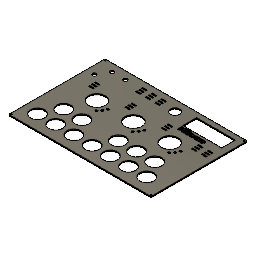
ArpeggioCase (Autodesk Fusion 360 design; units mm, degrees)
Autodesk Fusion 360 part; units mm, degrees
note: some values were not read from the file. Chosen so that the rebuilt part matches the saved one: a direction.
sketch "Sketch1" plane through (0, 0, 0) normal (0, 1, 0) x (1, 0, 0) in component "box"
  line L0 (130, 90) -> (-130, 90)
  line L1 (-130, 90) -> (-130, -90)
  line L2 (-130, -90) -> (130, -90)
  line L3 (130, -90) -> (130, 90)
  line L4 (130, 90) -> (-130, -90) construction
  line L5 (-130, 90) -> (130, -90) construction
  dimension "d1" = 260
  dimension "d2" = 180
extrude "Extrude1" add sketch "Sketch1" along normal blind 2 in component "box"
sketch "Sketch2" plane through (0, 2, 0) normal (0, 1, 0) x (-1, 0, 0) in component "box"
  line L0 (-130, 90) -> (-130, -90)
  line L1 (-130, -90) -> (130, -90)
  line L2 (130, -90) -> (130, 90)
  line L3 (130, 90) -> (-130, 90)
  circle A0 centre (107, 62) radius 13
  circle A1 centre (107, 62) radius 13
  circle A2 centre (73, 62) radius 13
  circle A3 centre (39, 62) radius 13
  circle A4 centre (5, 62) radius 13
  circle A5 centre (-29, 62) radius 13
  circle A6 centre (-63, 62) radius 13
  circle A7 centre (-97, 62) radius 13
  circle A8 centre (90, 30) radius 13
  circle A9 centre (56, 30) radius 13
  circle A10 centre (-12, 30) radius 13
  circle A11 centre (-46, 30) radius 13
  circle A12 centre (-80, 30) radius 13
  circle A13 centre (73, -15) radius 15.5
  circle A14 centre (73, -15) radius 15.5
  circle A15 centre (5, -15) radius 15.5
  circle A16 centre (-63, -15) radius 15.5
  line L4 (-120, -55) -> (-48, -55)
  line L5 (-48, -55) -> (-48, -80)
  line L6 (-48, -80) -> (-120, -80)
  line L7 (-120, -80) -> (-120, -55)
  line L8 (-120, -55) -> (-48, -80) construction
  line L9 (-48, -55) -> (-120, -80) construction
  circle A17 centre (105, -75) radius 3.5
  circle A18 centre (80, -75) radius 3.5
  circle A19 centre (-18, -70) radius 8.5
  dimension "d5" = 26
  dimension "d10" = 23
  dimension "d11" = 28
  dimension "d12" = 26
  dimension "d13" = 26
  dimension "d14" = 26
  dimension "d15" = 26
  dimension "d16" = 26
  dimension "d17" = 26
  dimension "d18" = 26
  dimension "d33" = 26
  dimension "d34" = 40
  dimension "d35" = 60
  dimension "d36" = 26
  dimension "d37" = 26
  dimension "d38" = 26
  dimension "d39" = 26
  dimension "d41" = 31
  dimension "d42" = 34
  dimension "d43" = 34
  dimension "d44" = 34
  dimension "d45" = 34
  dimension "d46" = 34
  dimension "d47" = 34
  dimension "d48" = 45
  dimension "d49" = 31
  dimension "d50" = 31
  dimension "d51" = 31
  dimension "d52" = 72
  dimension "d53" = 25
  dimension "d54" = 10
  dimension "d55" = 10
  dimension "d56" = 7
  dimension "d57" = 25
  dimension "d58" = 15
  dimension "d59" = 7
  dimension "d60" = 25
  dimension "d62" = 17
  dimension "d63" = 30
  dimension "d64" = 20
  measures "d5" diameter of A0
  measures "d12" diameter of A1
  measures "d13" diameter of A2
  measures "d14" diameter of A3
  measures "d15" diameter of A4
  measures "d16" diameter of A5
  measures "d17" diameter of A6
  measures "d18" diameter of A7
  measures "d33" diameter of A8
  measures "d36" diameter of A9
  measures "d37" diameter of A10
  measures "d38" diameter of A11
  measures "d39" diameter of A12
  measures "d41" diameter of A13
  measures "d44" distance of origin
  measures "d45" distance of origin
  measures "d48" distance of origin
  measures "d49" diameter of A14
  measures "d50" diameter of A15
  measures "d51" diameter of A16
  measures "d54" distance of L0 L7
  measures "d55" distance of L1 L6
  measures "d56" diameter of A17
  measures "d59" diameter of A18
  measures "d62" diameter of A19
extrude "Extrude9" cut sketch "Sketch2" against normal blind 2 contours A0 A1 | A2 | A3 | A4 | A5 | A6 | A7 | A8 | A9 | A10 | A11 | A12 | A13 A14 | A15 | A16 | L4 L5 L6 L7 | A17 | A18 | A19 in component "box"
sketch "Sketch1 (2)" plane through (0, 2, 0) normal (0, 1, 0) x (-1, 0, 0)
  line L0 (-48, -55) -> (-48, -80)
  line L1 (-48, -80) -> (-120, -80)
  line L2 (-120, -80) -> (-120, -55)
  line L3 (-120, -55) -> (-48, -55)
  circle A0 centre (73, -15) radius 15.5
  circle A1 centre (56, 30) radius 13
  circle A2 centre (-29, 62) radius 13
  circle A3 centre (107, 62) radius 13
  circle A4 centre (5, 62) radius 13
  circle A5 centre (90, 30) radius 13
  circle A6 centre (-80, 30) radius 13
  circle A7 centre (-18, -70) radius 8.5
  circle A8 centre (80, -75) radius 3.5
  circle A9 centre (5, -15) radius 15.5
  circle A10 centre (-12, 30) radius 13
  circle A11 centre (-63, 62) radius 13
  circle A12 centre (73, 62) radius 13
  circle A13 centre (39, 62) radius 13
  circle A14 centre (-97, 62) radius 13
  circle A15 centre (-46, 30) radius 13
  circle A16 centre (-63, -15) radius 15.5
  circle A17 centre (105, -75) radius 3.5
  line L4 (130, -90) -> (130, 90)
  line L5 (130, 90) -> (-130, 90)
  line L6 (-130, 90) -> (-130, -90)
  line L7 (-130, -90) -> (130, -90)
  line L8 (96, -43.5014) -> (104, -43.5014)
  line L9 (104, -43.5014) -> (104, -41.5014)
  line L10 (104, -41.5014) -> (96, -41.5014)
  line L11 (96, -41.5014) -> (96, -43.5014)
  line L12 (96, -43.5014) -> (104, -41.5014) construction
  line L13 (104, -43.5014) -> (96, -41.5014) construction
  line L14 (96, -32.5014) -> (104, -32.5014)
  line L15 (104, -32.5014) -> (104, -30.5014)
  line L16 (96, -30.5014) -> (96, -32.5014)
  line L17 (104, -30.5014) -> (96, -30.5014)
  line L18 (96, -32.5014) -> (104, -30.5014) construction
  line L19 (104, -32.5014) -> (96, -30.5014) construction
  line L20 (96, -36.0014) -> (96, -38.0014)
  line L21 (104, -38.0014) -> (96, -36.0014) construction
  line L22 (104, -36.0014) -> (96, -36.0014)
  line L23 (96, -38.0014) -> (104, -38.0014)
  line L24 (96, -38.0014) -> (104, -36.0014) construction
  line L25 (104, -38.0014) -> (104, -36.0014)
  line L26 (28, -38.0014) -> (36, -38.0014)
  line L27 (36, -30.5014) -> (28, -30.5014)
  line L28 (36, -38.0014) -> (36, -36.0014)
  line L29 (28, -43.5014) -> (36, -41.5014) construction
  line L30 (28, -32.5014) -> (36, -30.5014) construction
  line L31 (36, -32.5014) -> (28, -30.5014) construction
  line L32 (28, -36.0014) -> (28, -38.0014)
  line L33 (28, -30.5014) -> (28, -32.5014)
  line L34 (36, -43.5014) -> (36, -41.5014)
  line L35 (36, -43.5014) -> (28, -41.5014) construction
  line L36 (28, -38.0014) -> (36, -36.0014) construction
  line L37 (36, -32.5014) -> (36, -30.5014)
  line L38 (36, -41.5014) -> (28, -41.5014)
  line L39 (36, -38.0014) -> (28, -36.0014) construction
  line L40 (28, -32.5014) -> (36, -32.5014)
  line L41 (28, -43.5014) -> (36, -43.5014)
  line L42 (36, -36.0014) -> (28, -36.0014)
  line L43 (28, -41.5014) -> (28, -43.5014)
  line L44 (-32, -38.0014) -> (-32, -36.0014)
  line L45 (-40, -43.5014) -> (-32, -43.5014)
  line L46 (-40, -32.5014) -> (-32, -32.5014)
  line L47 (-32, -38.0014) -> (-40, -36.0014) construction
  line L48 (-40, -43.5014) -> (-32, -41.5014) construction
  line L49 (-32, -30.5014) -> (-40, -30.5014)
  line L50 (-40, -38.0014) -> (-32, -38.0014)
  line L51 (-40, -38.0014) -> (-32, -36.0014) construction
  line L52 (-40, -30.5014) -> (-40, -32.5014)
  line L53 (-32, -32.5014) -> (-32, -30.5014)
  line L54 (-40, -32.5014) -> (-32, -30.5014) construction
  line L55 (-32, -43.5014) -> (-32, -41.5014)
  line L56 (-32, -41.5014) -> (-40, -41.5014)
  line L57 (-40, -41.5014) -> (-40, -43.5014)
  line L58 (-32, -43.5014) -> (-40, -41.5014) construction
  line L59 (-32, -36.0014) -> (-40, -36.0014)
  line L60 (-32, -32.5014) -> (-40, -30.5014) construction
  line L61 (-40, -36.0014) -> (-40, -38.0014)
  circle A18 centre (48.684, -11.0058) radius 2
  circle A19 centre (52, -4) radius 2
  circle A20 centre (57, 2) radius 2
  circle A21 centre (-16, -4) radius 2
  circle A22 centre (-11, 2) radius 2
  circle A23 centre (-19.316, -11.0058) radius 2
  circle A24 centre (-87.316, -11.0058) radius 2
  circle A25 centre (-84, -4) radius 2
  circle A26 centre (-79, 2) radius 2
  line L62 (-120, -27.5014) -> (-112, -25.5014) construction
  line L63 (-112, -38.5014) -> (-120, -36.5014) construction
  line L64 (-112, -31.0014) -> (-120, -31.0014)
  line L65 (-112, -36.5014) -> (-120, -36.5014)
  line L66 (-112, -27.5014) -> (-112, -25.5014)
  line L67 (-112, -38.5014) -> (-112, -36.5014)
  line L68 (-112, -27.5014) -> (-120, -25.5014) construction
  line L69 (-120, -36.5014) -> (-120, -38.5014)
  line L70 (-120, -33.0014) -> (-112, -31.0014) construction
  line L71 (-120, -27.5014) -> (-112, -27.5014)
  line L72 (-120, -38.5014) -> (-112, -36.5014) construction
  line L73 (-112, -33.0014) -> (-120, -31.0014) construction
  line L74 (-120, -25.5014) -> (-120, -27.5014)
  line L75 (-120, -31.0014) -> (-120, -33.0014)
  line L76 (-112, -33.0014) -> (-112, -31.0014)
  line L77 (-112, -25.5014) -> (-120, -25.5014)
  line L78 (-120, -38.5014) -> (-112, -38.5014)
  line L79 (-120, -33.0014) -> (-112, -33.0014)
  line L80 (-101.4634, -27.3193) -> (-93.4634, -27.3193)
  line L81 (-101.4634, -25.3193) -> (-101.4634, -27.3193)
  line L82 (-93.4634, -36.3193) -> (-101.4634, -36.3193)
  line L83 (-101.4634, -36.3193) -> (-101.4634, -38.3193)
  line L84 (-93.4634, -38.3193) -> (-101.4634, -36.3193) construction
  line L85 (-93.4634, -30.8193) -> (-101.4634, -30.8193)
  line L86 (-93.4634, -27.3193) -> (-101.4634, -25.3193) construction
  line L87 (-101.4634, -32.8193) -> (-93.4634, -30.8193) construction
  line L88 (-93.4634, -25.3193) -> (-101.4634, -25.3193)
  line L89 (-101.4634, -38.3193) -> (-93.4634, -36.3193) construction
  line L90 (-101.4634, -30.8193) -> (-101.4634, -32.8193)
  line L91 (-101.4634, -27.3193) -> (-93.4634, -25.3193) construction
  line L92 (-93.4634, -27.3193) -> (-93.4634, -25.3193)
  line L93 (-93.4634, -38.3193) -> (-93.4634, -36.3193)
  line L94 (-93.4634, -32.8193) -> (-93.4634, -30.8193)
  line L95 (-101.4634, -38.3193) -> (-93.4634, -38.3193)
  line L96 (-93.4634, -32.8193) -> (-101.4634, -30.8193) construction
  line L97 (-101.4634, -32.8193) -> (-93.4634, -32.8193)
  line L98 (43, -73.0014) -> (51, -73.0014)
  line L99 (51, -67.5014) -> (43, -65.5014) construction
  line L100 (51, -71.0014) -> (43, -71.0014)
  line L101 (51, -76.5014) -> (43, -76.5014)
  line L102 (43, -76.5014) -> (43, -78.5014)
  line L103 (43, -65.5014) -> (43, -67.5014)
  line L104 (43, -73.0014) -> (51, -71.0014) construction
  line L105 (51, -67.5014) -> (51, -65.5014)
  line L106 (43, -67.5014) -> (51, -67.5014)
  line L107 (51, -73.0014) -> (51, -71.0014)
  line L108 (51, -65.5014) -> (43, -65.5014)
  line L109 (43, -71.0014) -> (43, -73.0014)
  line L110 (51, -78.5014) -> (51, -76.5014)
  line L111 (43, -78.5014) -> (51, -78.5014)
  line L112 (51, -78.5014) -> (43, -76.5014) construction
  line L113 (43, -78.5014) -> (51, -76.5014) construction
  line L114 (43, -67.5014) -> (51, -65.5014) construction
  line L115 (51, -73.0014) -> (43, -71.0014) construction
  line L116 (25, -65.5014) -> (25, -67.5014)
  line L117 (25, -73.0014) -> (33, -73.0014)
  line L118 (33, -71.0014) -> (25, -71.0014)
  line L119 (33, -76.5014) -> (25, -76.5014)
  line L120 (33, -67.5014) -> (25, -65.5014) construction
  line L121 (25, -76.5014) -> (25, -78.5014)
  line L122 (25, -73.0014) -> (33, -71.0014) construction
  line L123 (33, -67.5014) -> (33, -65.5014)
  line L124 (25, -67.5014) -> (33, -67.5014)
  line L125 (25, -78.5014) -> (33, -78.5014)
  line L126 (25, -78.5014) -> (33, -76.5014) construction
  line L127 (33, -78.5014) -> (25, -76.5014) construction
  line L128 (25, -67.5014) -> (33, -65.5014) construction
  line L129 (33, -73.0014) -> (25, -71.0014) construction
  line L130 (33, -73.0014) -> (33, -71.0014)
  line L131 (33, -65.5014) -> (25, -65.5014)
  line L132 (33, -78.5014) -> (33, -76.5014)
  line L133 (25, -71.0014) -> (25, -73.0014)
  line L134 (7, -67.5014) -> (15, -65.5014) construction
  line L135 (7, -67.5014) -> (15, -67.5014)
  line L136 (15, -65.5014) -> (7, -65.5014)
  line L137 (7, -73.0014) -> (15, -73.0014)
  line L138 (7, -71.0014) -> (7, -73.0014)
  line L139 (15, -71.0014) -> (7, -71.0014)
  line L140 (15, -76.5014) -> (7, -76.5014)
  line L141 (7, -73.0014) -> (15, -71.0014) construction
  line L142 (15, -78.5014) -> (15, -76.5014)
  line L143 (15, -67.5014) -> (15, -65.5014)
  line L144 (15, -73.0014) -> (7, -71.0014) construction
  line L145 (7, -78.5014) -> (15, -76.5014) construction
  line L146 (7, -78.5014) -> (15, -78.5014)
  line L147 (15, -78.5014) -> (7, -76.5014) construction
  line L148 (15, -73.0014) -> (15, -71.0014)
  line L149 (7, -65.5014) -> (7, -67.5014)
  line L150 (7, -76.5014) -> (7, -78.5014)
  line L151 (15, -67.5014) -> (7, -65.5014) construction
  dimension "d67" = 8
  dimension "d68" = 2
  dimension "d69" = 8
  dimension "d70" = 2
  dimension "d71" = 13
  dimension "d72" = 8
  dimension "d73" = 2
  dimension "d74" = 6.5
  dimension "d75" = 8
  dimension "d76" = 2
  dimension "d77" = 8
  dimension "d78" = 2
  dimension "d79" = 13
  dimension "d80" = 8
  dimension "d81" = 2
  dimension "d82" = 6.5
  dimension "d83" = 8
  dimension "d84" = 2
  dimension "d85" = 8
  dimension "d86" = 2
  dimension "d87" = 13
  dimension "d88" = 8
  dimension "d89" = 2
  dimension "d90" = 6.5
  dimension "d92" = 23
  dimension "d93" = 23
  dimension "d94" = 23
  dimension "d97" = 4
  dimension "d98" = 4
  dimension "d99" = 4
  dimension "d100" = 4
  dimension "d101" = 4
  dimension "d102" = 4
  dimension "d103" = 4
  dimension "d104" = 4
  dimension "d105" = 4
  dimension "d106" = 8
  dimension "d107" = 2
  dimension "d108" = 8
  dimension "d109" = 2
  dimension "d110" = 13
  dimension "d111" = 8
  dimension "d112" = 2
  dimension "d113" = 6.5
  dimension "d114" = 8
  dimension "d115" = 2
  dimension "d116" = 8
  dimension "d117" = 2
  dimension "d118" = 13
  dimension "d119" = 8
  dimension "d120" = 2
  dimension "d121" = 6.5
  dimension "d122" = 8
  dimension "d123" = 2
  dimension "d124" = 8
  dimension "d125" = 2
  dimension "d126" = 13
  dimension "d127" = 8
  dimension "d128" = 2
  dimension "d129" = 6.5
  dimension "d130" = 8
  dimension "d131" = 2
  dimension "d132" = 8
  dimension "d133" = 2
  dimension "d134" = 13
  dimension "d135" = 8
  dimension "d136" = 2
  dimension "d137" = 6.5
  dimension "d138" = 8
  dimension "d139" = 2
  dimension "d140" = 8
  dimension "d141" = 2
  dimension "d142" = 13
  dimension "d143" = 8
  dimension "d144" = 2
  dimension "d145" = 6.5
  dimension "d146" = 10
  dimension "d147" = 10
  measures "d92" distance of origin
  measures "d93" distance of origin
  measures "d94" distance of origin
  measures "d97" diameter of A18
  measures "d98" diameter of A19
  measures "d99" diameter of A20
  measures "d100" diameter of A23
  measures "d101" diameter of A21
  measures "d102" diameter of A22
  measures "d103" diameter of A24
  measures "d104" diameter of A25
  measures "d105" diameter of A26
  measures "d147" distance of origin
extrude "Extrude10" cut sketch "Sketch1 (2)" against normal blind 2 contours L8 L9 L10 L11 | L14 L15 L16 L17 | L20 L22 L23 L25 | L26 L28 L32 L42 | L27 L33 L37 L40 | L34 L38 L41 L43 | L44 L50 L59 L61 | L45 L55 L56 L57 | L46 L49 L52 L53 | A18 | A19 | A20 | A21 | A22 | A23 | A24 | A25 | A26 | L64 L75 L76 L79 | L65 L67 L69 L78 | L66 L71 L74 L77 | L80 L81 L88 L92 | L82 L83 L93 L95 | L85 L90 L94 L97 | L98 L100 L107 L109 | L101 L102 L110 L111 | L103 L105 L106 L108 | L116 L123 L124 L131 | L117 L118 L130 L133 | L119 L121 L125 L132 | L135 L136 L143 L149 | L137 L138 L139 L148 | L140 L142 L146 L150 in component "box"
extrude "Extrude11" add 1 faces at (130, 0.6667, 30) along direction (1, 0, 0) blind 3 in component "box"
extrude "Extrude12" add 1 faces at (-130, 0.6667, -30) along direction (-1, 0, 0) blind 3 in component "box"
hole "Hole1" at (-130, 2, 87) direction (0, -1, 0) diameter 1.875 depth 2 tip angle 118 in component "box"
thread "Thread1" "ISO Metric profile 2.3 M2.3x0.45 6H" in component "box"
pattern_linear "R-Pattern1" count 2 spacing 174 along (0, 0, -1) count 2 spacing 260 along (1, 0, 0) of "Hole1" in component "box"
sketch "Sketch2 (2)" plane through (0, 37.5554, 0) normal (0, 1, 0) x (-1, 0, 0)
  circle A0 centre (-43.4219, 26.2013) radius 0.9377
  circle A1 centre (-43.4219, 200.2013) radius 0.9377
  circle A2 centre (216.5781, 26.2013) radius 0.9377
  circle A3 centre (216.5781, 200.2013) radius 0.9377
  line L0 (101.5781, 45.6998) -> (93.5781, 45.6998)
  line L1 (93.5781, 45.6998) -> (93.5781, 47.6998)
  line L2 (93.5781, 47.6998) -> (101.5781, 47.6998)
  line L3 (101.5781, 47.6998) -> (101.5781, 45.6998)
  circle A4 centre (7.5781, 115.2013) radius 2
  circle A5 centre (138.5781, 109.2013) radius 2
  circle A6 centre (67.2621, 102.1955) radius 2
  line L4 (-14.8853, 87.8819) -> (-6.8853, 87.8819)
  line L5 (-6.8853, 87.8819) -> (-6.8853, 85.8819)
  line L6 (-6.8853, 85.8819) -> (-14.8853, 85.8819)
  line L7 (-14.8853, 85.8819) -> (-14.8853, 87.8819)
  line L8 (137.5781, 40.1998) -> (129.5781, 40.1998)
  line L9 (129.5781, 40.1998) -> (129.5781, 42.1998)
  line L10 (129.5781, 42.1998) -> (137.5781, 42.1998)
  line L11 (137.5781, 42.1998) -> (137.5781, 40.1998)
  line L12 (54.5781, 69.6998) -> (46.5781, 69.6998)
  line L13 (46.5781, 69.6998) -> (46.5781, 71.6998)
  line L14 (46.5781, 71.6998) -> (54.5781, 71.6998)
  line L15 (54.5781, 71.6998) -> (54.5781, 69.6998)
  line L16 (190.5781, 69.6998) -> (182.5781, 69.6998)
  line L17 (182.5781, 69.6998) -> (182.5781, 71.6998)
  line L18 (182.5781, 71.6998) -> (190.5781, 71.6998)
  line L19 (190.5781, 71.6998) -> (190.5781, 69.6998)
  line L20 (182.5781, 77.1998) -> (190.5781, 77.1998)
  line L21 (190.5781, 77.1998) -> (190.5781, 75.1998)
  line L22 (190.5781, 75.1998) -> (182.5781, 75.1998)
  line L23 (182.5781, 75.1998) -> (182.5781, 77.1998)
  line L24 (122.5781, 69.6998) -> (114.5781, 69.6998)
  line L25 (114.5781, 69.6998) -> (114.5781, 71.6998)
  line L26 (114.5781, 71.6998) -> (122.5781, 71.6998)
  line L27 (122.5781, 71.6998) -> (122.5781, 69.6998)
  line L28 (137.5781, 36.6998) -> (137.5781, 34.6998)
  line L29 (137.5781, 34.6998) -> (129.5781, 34.6998)
  line L30 (129.5781, 34.6998) -> (129.5781, 36.6998)
  line L31 (129.5781, 36.6998) -> (137.5781, 36.6998)
  line L32 (-6.8852, 82.3819) -> (-6.8852, 80.3819)
  line L33 (-6.8852, 80.3819) -> (-14.8852, 80.3819)
  line L34 (-14.8852, 80.3819) -> (-14.8852, 82.3819)
  line L35 (-14.8852, 82.3819) -> (-6.8852, 82.3819)
  line L36 (-25.4219, 76.6998) -> (-25.4219, 74.6998)
  line L37 (-25.4219, 74.6998) -> (-33.4219, 74.6998)
  line L38 (-33.4219, 74.6998) -> (-33.4219, 76.6998)
  line L39 (-33.4219, 76.6998) -> (-25.4219, 76.6998)
  circle A7 centre (143.5781, 115.2013) radius 2
  circle A8 centre (2.5781, 109.2013) radius 2
  line L40 (111.5781, 45.6998) -> (111.5781, 47.6998)
  line L41 (111.5781, 47.6998) -> (119.5781, 47.6998)
  line L42 (119.5781, 47.6998) -> (119.5781, 45.6998)
  line L43 (119.5781, 45.6998) -> (111.5781, 45.6998)
  line L44 (93.5781, 42.1998) -> (101.5781, 42.1998)
  line L45 (101.5781, 42.1998) -> (101.5781, 40.1998)
  line L46 (101.5781, 40.1998) -> (93.5781, 40.1998)
  line L47 (93.5781, 40.1998) -> (93.5781, 42.1998)
  line L48 (111.5781, 36.6998) -> (119.5781, 36.6998)
  line L49 (119.5781, 36.6998) -> (119.5781, 34.6998)
  line L50 (119.5781, 34.6998) -> (111.5781, 34.6998)
  line L51 (111.5781, 34.6998) -> (111.5781, 36.6998)
  circle A9 centre (135.2621, 102.1955) radius 2
  circle A10 centre (70.5781, 109.2013) radius 2
  line L52 (-33.4219, 85.6998) -> (-33.4219, 87.6998)
  line L53 (-33.4219, 87.6998) -> (-25.4219, 87.6998)
  line L54 (-25.4219, 87.6998) -> (-25.4219, 85.6998)
  line L55 (-25.4219, 85.6998) -> (-33.4219, 85.6998)
  line L56 (129.5781, 45.6998) -> (129.5781, 47.6998)
  line L57 (129.5781, 47.6998) -> (137.5781, 47.6998)
  line L58 (137.5781, 47.6998) -> (137.5781, 45.6998)
  line L59 (137.5781, 45.6998) -> (129.5781, 45.6998)
  line L60 (54.5781, 75.1998) -> (46.5781, 75.1998)
  line L61 (46.5781, 75.1998) -> (46.5781, 77.1998)
  line L62 (46.5781, 77.1998) -> (54.5781, 77.1998)
  line L63 (54.5781, 77.1998) -> (54.5781, 75.1998)
  line L64 (122.5781, 82.6998) -> (122.5781, 80.6998)
  line L65 (122.5781, 80.6998) -> (114.5781, 80.6998)
  line L66 (114.5781, 80.6998) -> (114.5781, 82.6998)
  line L67 (114.5781, 82.6998) -> (122.5781, 82.6998)
  line L68 (182.5781, 80.6998) -> (182.5781, 82.6998)
  line L69 (182.5781, 82.6998) -> (190.5781, 82.6998)
  line L70 (190.5781, 82.6998) -> (190.5781, 80.6998)
  line L71 (190.5781, 80.6998) -> (182.5781, 80.6998)
  line L72 (114.5781, 75.1998) -> (114.5781, 77.1998)
  line L73 (114.5781, 77.1998) -> (122.5781, 77.1998)
  line L74 (122.5781, 77.1998) -> (122.5781, 75.1998)
  line L75 (122.5781, 75.1998) -> (114.5781, 75.1998)
  line L76 (46.5781, 82.6998) -> (54.5781, 82.6998)
  line L77 (54.5781, 82.6998) -> (54.5781, 80.6998)
  line L78 (54.5781, 80.6998) -> (46.5781, 80.6998)
  line L79 (46.5781, 80.6998) -> (46.5781, 82.6998)
  line L80 (-6.8852, 76.8819) -> (-6.8852, 74.8819)
  line L81 (-6.8852, 74.8819) -> (-14.8852, 74.8819)
  line L82 (-14.8852, 74.8819) -> (-14.8852, 76.8819)
  line L83 (-14.8852, 76.8819) -> (-6.8852, 76.8819)
  line L84 (-25.4219, 82.1998) -> (-25.4219, 80.1998)
  line L85 (-25.4219, 80.1998) -> (-33.4219, 80.1998)
  line L86 (-33.4219, 80.1998) -> (-33.4219, 82.1998)
  line L87 (-33.4219, 82.1998) -> (-25.4219, 82.1998)
  circle A11 centre (75.5781, 115.2013) radius 2
  circle A12 centre (-0.7379, 102.1955) radius 2
  line L88 (119.5781, 40.1998) -> (111.5781, 40.1998)
  line L89 (111.5781, 40.1998) -> (111.5781, 42.1998)
  line L90 (111.5781, 42.1998) -> (119.5781, 42.1998)
  line L91 (119.5781, 42.1998) -> (119.5781, 40.1998)
  line L92 (101.5781, 34.6998) -> (93.5781, 34.6998)
  line L93 (93.5781, 34.6998) -> (93.5781, 36.6998)
  line L94 (93.5781, 36.6998) -> (101.5781, 36.6998)
  line L95 (101.5781, 36.6998) -> (101.5781, 34.6998)
  line L96 (38.5781, 58.2013) -> (38.5781, 33.2013)
  line L97 (38.5781, 33.2013) -> (-33.4219, 33.2013)
  line L98 (-33.4219, 33.2013) -> (-33.4219, 58.2013)
  line L99 (-33.4219, 58.2013) -> (38.5781, 58.2013)
  circle A13 centre (159.5781, 98.2013) radius 15.5
  circle A14 centre (142.5781, 143.2013) radius 13
  circle A15 centre (57.5781, 175.2013) radius 13
  circle A16 centre (193.5781, 175.2013) radius 13
  circle A17 centre (91.5781, 175.2013) radius 13
  circle A18 centre (176.5781, 143.2013) radius 13
  circle A19 centre (6.5781, 143.2013) radius 13
  circle A20 centre (68.5781, 43.2013) radius 8.5
  circle A21 centre (166.5781, 38.2013) radius 3.5
  circle A22 centre (91.5781, 98.2013) radius 15.5
  circle A23 centre (74.5781, 143.2013) radius 13
  circle A24 centre (23.5781, 175.2013) radius 13
  circle A25 centre (159.5781, 175.2013) radius 13
  circle A26 centre (125.5781, 175.2013) radius 13
  circle A27 centre (-10.4219, 175.2013) radius 13
  circle A28 centre (40.5781, 143.2013) radius 13
  circle A29 centre (23.5781, 98.2013) radius 15.5
  circle A30 centre (191.5781, 38.2013) radius 3.5
  line L100 (-46.4219, 23.2013) -> (219.5781, 23.2013)
  line L101 (219.5781, 23.2013) -> (219.5781, 203.2013)
  line L102 (219.5781, 203.2013) -> (-46.4219, 203.2013)
  line L103 (-46.4219, 203.2013) -> (-46.4219, 23.2013)
hole "Hole2" at (-117.509, 2, -54.652) direction (0, -1, 0) diameter 7 depth 2 tip angle 118 in component "box"
fillet "Fillet2" radius 2 4 edges at (133, 1, -90) (-133, 1, -90) (133, 1, 90) (-133, 1, 90) in component "box"
sketch "Sketch4" plane through (-86.5781, 37.5554, 113.2013) normal (0, 1, 0) x (-1, 0, 0)
  line L0 (-51.7625, -43.625) -> (-49.3426, -43.625)
  line L1 (-49.3426, -43.625) -> (-49.3426, -52.0947)
  line L2 (-49.3426, -52.0947) -> (-51.7625, -52.0947)
  line L3 (-51.7625, -52.0947) -> (-51.7625, -50.8847)
  line L4 (-51.7625, -50.8847) -> (-52.9725, -50.8847)
  line L5 (-52.9725, -50.8847) -> (-52.9725, -49.6748)
  line L6 (-52.9725, -49.6748) -> (-54.1824, -49.6748)
  line L7 (-54.1824, -49.6748) -> (-54.1824, -50.8847)
  line L8 (-54.1824, -50.8847) -> (-55.3924, -50.8847)
  line L9 (-55.3924, -50.8847) -> (-55.3924, -52.0947)
  line L10 (-55.3924, -52.0947) -> (-57.8123, -52.0947)
  line L11 (-57.8123, -52.0947) -> (-57.8123, -43.625)
  line L12 (-57.8123, -43.625) -> (-55.3924, -43.625)
  line L13 (-55.3924, -43.625) -> (-55.3924, -48.4648)
  line L14 (-55.3924, -48.4648) -> (-54.1824, -48.4648)
  line L15 (-54.1824, -48.4648) -> (-54.1824, -46.0449)
  line L16 (-54.1824, -46.0449) -> (-52.9725, -46.0449)
  line L17 (-52.9725, -46.0449) -> (-52.9725, -48.4648)
  line L18 (-52.9725, -48.4648) -> (-51.7625, -48.4648)
  line L19 (-51.7625, -48.4648) -> (-51.7625, -43.625)
  line L20 (-61.4422, -43.625) -> (-59.0223, -43.625)
  line L21 (-59.0223, -43.625) -> (-59.0223, -52.0947)
  line L22 (-59.0223, -52.0947) -> (-66.282, -52.0947)
  line L23 (-66.282, -52.0947) -> (-66.282, -50.8847)
  line L24 (-66.282, -50.8847) -> (-67.4919, -50.8847)
  line L25 (-67.4919, -50.8847) -> (-67.4919, -47.2549)
  line L26 (-67.4919, -47.2549) -> (-65.072, -47.2549)
  line L27 (-65.072, -47.2549) -> (-65.072, -46.0449)
  line L28 (-65.072, -46.0449) -> (-66.282, -46.0449)
  line L29 (-66.282, -46.0449) -> (-66.282, -44.835)
  line L30 (-66.282, -44.835) -> (-67.4919, -44.835)
  line L31 (-67.4919, -44.835) -> (-67.4919, -43.625)
  line L32 (-67.4919, -43.625) -> (-63.8621, -43.625)
  line L33 (-63.8621, -43.625) -> (-63.8621, -44.835)
  line L34 (-63.8621, -44.835) -> (-62.6521, -44.835)
  line L35 (-62.6521, -44.835) -> (-62.6521, -46.0449)
  line L36 (-62.6521, -46.0449) -> (-61.4422, -46.0449)
  line L37 (-61.4422, -46.0449) -> (-61.4422, -43.625)
  line L38 (-61.4422, -50.8847) -> (-61.4422, -47.2549)
  line L39 (-61.4422, -47.2549) -> (-63.8621, -47.2549)
  line L40 (-63.8621, -47.2549) -> (-63.8621, -48.4648)
  line L41 (-63.8621, -48.4648) -> (-65.072, -48.4648)
  line L42 (-65.072, -48.4648) -> (-65.072, -50.8847)
  line L43 (-65.072, -50.8847) -> (-61.4422, -50.8847)
  line L44 (-75.9616, -43.625) -> (-69.9118, -43.625)
  line L45 (-69.9118, -43.625) -> (-69.9118, -44.835)
  line L46 (-69.9118, -44.835) -> (-68.7019, -44.835)
  line L47 (-68.7019, -44.835) -> (-68.7019, -48.4648)
  line L48 (-68.7019, -48.4648) -> (-69.9118, -48.4648)
  line L49 (-69.9118, -48.4648) -> (-69.9118, -49.6748)
  line L50 (-69.9118, -49.6748) -> (-75.9616, -49.6748)
  line L51 (-75.9616, -49.6748) -> (-75.9616, -48.4648)
  line L52 (-75.9616, -48.4648) -> (-77.1715, -48.4648)
  line L53 (-77.1715, -48.4648) -> (-77.1715, -44.835)
  line L54 (-77.1715, -44.835) -> (-75.9616, -44.835)
  line L55 (-75.9616, -44.835) -> (-75.9616, -43.625)
  line L56 (-71.1218, -48.4648) -> (-71.1218, -44.835)
  line L57 (-71.1218, -44.835) -> (-74.7516, -44.835)
  line L58 (-74.7516, -44.835) -> (-74.7516, -48.4648)
  line L59 (-74.7516, -48.4648) -> (-71.1218, -48.4648)
  line L60 (-86.8511, -43.625) -> (-78.3815, -43.625)
  line L61 (-78.3815, -43.625) -> (-78.3815, -44.835)
  line L62 (-78.3815, -44.835) -> (-79.5914, -44.835)
  line L63 (-79.5914, -44.835) -> (-79.5914, -46.0449)
  line L64 (-79.5914, -46.0449) -> (-80.8014, -46.0449)
  line L65 (-80.8014, -46.0449) -> (-80.8014, -47.2549)
  line L66 (-80.8014, -47.2549) -> (-82.0113, -47.2549)
  line L67 (-82.0113, -47.2549) -> (-82.0113, -48.4648)
  line L68 (-82.0113, -48.4648) -> (-78.3815, -48.4648)
  line L69 (-78.3815, -48.4648) -> (-78.3815, -49.6748)
  line L70 (-78.3815, -49.6748) -> (-86.8511, -49.6748)
  line L71 (-86.8511, -49.6748) -> (-86.8511, -48.4648)
  line L72 (-86.8511, -48.4648) -> (-85.6412, -48.4648)
  line L73 (-85.6412, -48.4648) -> (-85.6412, -47.2549)
  line L74 (-85.6412, -47.2549) -> (-84.4312, -47.2549)
  line L75 (-84.4312, -47.2549) -> (-84.4312, -46.0449)
  line L76 (-84.4312, -46.0449) -> (-83.2213, -46.0449)
  line L77 (-83.2213, -46.0449) -> (-83.2213, -44.835)
  line L78 (-83.2213, -44.835) -> (-86.8511, -44.835)
  line L79 (-86.8511, -44.835) -> (-86.8511, -43.625)
  line L80 (-95.3208, -43.625) -> (-89.271, -43.625)
  line L81 (-89.271, -43.625) -> (-89.271, -44.835)
  line L82 (-89.271, -44.835) -> (-88.0611, -44.835)
  line L83 (-88.0611, -44.835) -> (-88.0611, -48.4648)
  line L84 (-88.0611, -48.4648) -> (-89.271, -48.4648)
  line L85 (-89.271, -48.4648) -> (-89.271, -49.6748)
  line L86 (-89.271, -49.6748) -> (-95.3208, -49.6748)
  line L87 (-95.3208, -49.6748) -> (-95.3208, -48.4648)
  line L88 (-95.3208, -48.4648) -> (-96.5307, -48.4648)
  line L89 (-96.5307, -48.4648) -> (-96.5307, -46.0449)
  line L90 (-96.5307, -46.0449) -> (-90.481, -46.0449)
  line L91 (-90.481, -46.0449) -> (-90.481, -44.835)
  line L92 (-90.481, -44.835) -> (-95.3208, -44.835)
  line L93 (-95.3208, -44.835) -> (-95.3208, -43.625)
  line L94 (-90.481, -48.4648) -> (-90.481, -47.2549)
  line L95 (-90.481, -47.2549) -> (-94.1108, -47.2549)
  line L96 (-94.1108, -47.2549) -> (-94.1108, -48.4648)
  line L97 (-94.1108, -48.4648) -> (-90.481, -48.4648)
extrude "Extrude13" add sketch "Sketch4" along normal blind 1 draft -20 sketch seen with x (1, 0, 0) y (0, 1, 0) z (0, 0, 1) at (86.5781, -35.5554, -113.2013) in component "box"
component "box" placed x (1, 0, 0) y (0, 1, 0) z (0, 0, 1) at (-86.5781, 35.5554, 113.2013)
